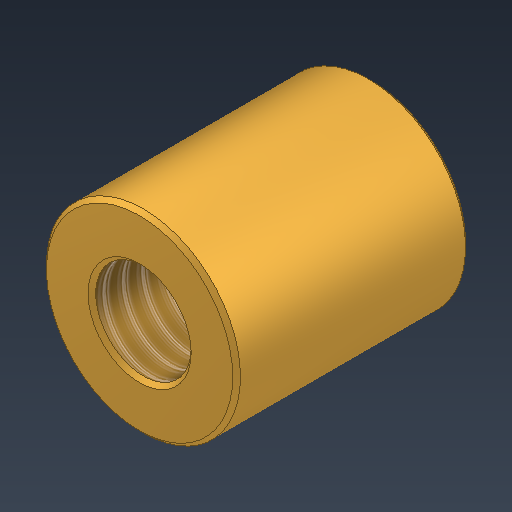
# Autodesk Inventor part: SB-305060
Saved by Autodesk Inventor 2021 (Build 250183000, 183)
## iProperties
Created: 2020-09-13
Part Number: SB-305060
Material: 真鍮、ソフト イエロー
Document SubType Name: Modeling
Designer: Yuta Kage
Mass: 0.628769 g
Surface Area: 1.44632 cm^2
Volume: 0.0742349 cm^3
Density: 8.47 g/cm^3
Appearance: 真鍮 - サテン
Description: 在庫有
購入先: ミスミ
在庫数: 15.0
Author: Yuta Kage
Autodesk Inventor part; units mm, degrees
ref_plane "YZ Plane" through (0, 0, 0) normal (1, 0, 0) x (0, 1, 0)
ref_plane "XZ Plane" through (0, 0, 0) normal (0, 1, 0) x (-1, 0, 0)
ref_plane "XY Plane" through (0, 0, 0) normal (0, 0, 1) x (1, 0, 0)
sketch "スケッチ1" plane through (0, 0, 0) normal (0, 0, 1) x (1, 0, 0)
  circle A0 centre (0, 0) radius 2.5
  dimension "d0" = 5
  constraints: 1 centre point, 1 coincident
  measures "d0" diameter of A0
extrude "押し出し1" add sketch "スケッチ1" along normal blind 6
sketch "スケッチ2" plane through (0, 0, 6) normal (0, 0, 1) x (1, 0, 0)
  circle A0 centre (0, 0) radius 2.5 construction
hole "穴1" at (0, 0, 6) direction (0, 0, -1) diameter 2.459 end through all thread size "M3x0.5" class "6H" standard "ANSI Metric M Profile"
chamfer "面取り1" distance 0.1 angle 45 4 edges at (0, 1.2295, 6) (-2.5, 0, 6) (-2.5, 0, 0) (0, 1.2295, 0)
